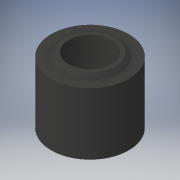
# Autodesk Inventor part: m5_9mm
Saved by Autodesk Inventor 2017 (Build 210142000, 142)
## iProperties
Created: 2016-08-18
Part Number: m5_9mm
Material: Generic
Document SubType Name: Modeling
Designer: brent
Density: 1 g/cm^3
Appearance: Default
Author: brent
Autodesk Inventor part; units mm, degrees
ref_plane "YZ Plane" through (0, 0, 0) normal (1, 0, 0) x (0, 1, 0)
ref_plane "XZ Plane" through (0, 0, 0) normal (0, 1, 0) x (-1, 0, 0)
ref_plane "XY Plane" through (0, 0, 0) normal (0, 0, 1) x (1, 0, 0)
sketch "Sketch1" plane through (0, 0, 0) normal (0, 1, 0) x (-1, 0, 0)
  circle A0 centre (0, 0) radius 2.75
  circle A1 centre (0, 0) radius 5
  dimension "d0" = 5.5
  dimension "d1" = 10
  constraints: 2 centre point, 2 coincident
  measures "d0" diameter of A0
  measures "d1" diameter of A1
extrude "Extrusion1" add sketch "Sketch1" along normal blind 8.5
sketch "Sketch2" plane through (0, 8.5, 0) normal (0, 1, 0) x (1, 0, 0)
  circle A0 centre (0, 0) radius 2.75 projected
  circle A1 centre (0, 0) radius 5 projected
  circle A2 centre (0, 0) radius 3.75
  dimension "d4" = 1
  constraints: 1 centre point, 1 coincident
  measures "d4" radial gap between concentric circles of A0 A2
extrude "Extrusion2" cut sketch "Sketch2" against normal blind 0.5 contours A1
chamfer "Chamfer1" distance 0.5 angle 45 1 edges at (-3.75, 8.5, 0)
body "Solid1"
